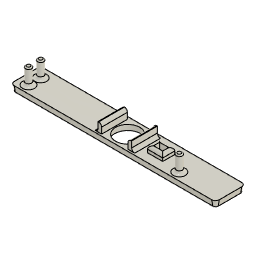
Front_Cover_OV5648_120DEG_AF v13 (Autodesk Fusion 360 design; units mm, degrees)
Autodesk Fusion 360 part; units mm, degrees
sketch "Sketch1" plane through (0, 0, 0) normal (0, 0, 1) x (1, 0, 0) in component "FrontCover"
  line L0 (0.9, 0) -> (66.1, 0)
  line L1 (67, 0.9) -> (67, 8.3)
  line L2 (66.1, 9.2) -> (0.9, 9.2)
  line L3 (0, 8.3) -> (0, 0.9)
  arc A0 (0.9, 9.2) -> (0, 8.3) centre (0.9, 8.3) ccw
  arc A1 (67, 8.3) -> (66.1, 9.2) centre (66.1, 8.3) ccw
  arc A2 (66.1, 0) -> (67, 0.9) centre (66.1, 0.9) ccw
  arc A3 (0, 0.9) -> (0.9, 0) centre (0.9, 0.9) ccw
  point P0 (67, 0)
  point P1 (0, 9.2)
  dimension "d1" = 67
  dimension "d2" = 9.2
  dimension "d3" = 0.9
  constraint horizontal L0
  constraint vertical L1
  constraint horizontal L2
  constraint vertical L3
  constraint coincident P1 L2
  constraint coincident P1 L3
  constraint tangent L2 A0
  constraint tangent L3 A0
  constraint tangent L1 A1
  constraint tangent L2 A1
  constraint equal A0 A1
  constraint coincident P0 L0
  constraint coincident P0 L1
  constraint tangent L0 A2
  constraint tangent L1 A2
  constraint equal A0 A2
  constraint coincident origin L0
  constraint coincident origin L3
  constraint tangent L0 A3
  constraint tangent L3 A3
  constraint equal A0 A3
  measures "d1" distance of origin P0
  measures "d2" distance of origin P1
  measures "d3" radius of A0
extrude "Extrude1" add sketch "Sketch1" along normal blind 2 draft 10 in component "FrontCover"
sketch "Sketch2" plane through (0, 0, 2) normal (0, 0, 1) x (-1, 0, 0) in component "FrontCover"
  line L0 (0.3527, -8.3) -> (0.3527, -0.9)
  arc A0 (0.3527, -0.9) -> (-0.9, 0.3527) centre (-0.9, -0.9) ccw
  line L1 (-0.9, 0.3527) -> (-66.1, 0.3527)
  arc A1 (-66.1, 0.3527) -> (-67.3527, -0.9) centre (-66.1, -0.9) ccw
  line L2 (-67.3527, -0.9) -> (-67.3527, -8.3)
  arc A2 (-67.3527, -8.3) -> (-66.1, -9.5527) centre (-66.1, -8.3) ccw
  line L3 (-66.1, -9.5527) -> (-0.9, -9.5527)
  arc A3 (-0.9, -9.5527) -> (0.3527, -8.3) centre (-0.9, -8.3) ccw
  line L4 (-66.1, -9.2) -> (-0.9, -9.2)
  arc A4 (-0.9, -9.2) -> (0, -8.3) centre (-0.9, -8.3) ccw
  line L5 (0, -8.3) -> (0, -0.9)
  arc A5 (0, -0.9) -> (-0.9, 0) centre (-0.9, -0.9) ccw
  line L6 (-0.9, 0) -> (-66.1, 0)
  arc A6 (-66.1, 0) -> (-67, -0.9) centre (-66.1, -0.9) ccw
  line L7 (-67, -0.9) -> (-67, -8.3)
  arc A7 (-67, -8.3) -> (-66.1, -9.2) centre (-66.1, -8.3) ccw
  line L8 (-1, -9.2) -> (-1, 0) construction
  circle A8 centre (-3, -6.25) radius 1
  circle A9 centre (-3, -2.25) radius 1
  circle A10 centre (-33.5, -4.5) radius 4
  circle A11 centre (-52.8, -2.25) radius 1
  line L9 (-37.85, -8.75) -> (-37.85, -0.25)
  line L10 (-29.15, -0.25) -> (-29.15, -8.75)
  line L11 (-29.15, -8.75) -> (-37.85, -0.25) construction
  line L12 (-37.85, -8.75) -> (-29.15, -0.25) construction
  line L13 (-27.95, -0.25) -> (-27.95, -8.75)
  line L14 (-39.05, -8.75) -> (-39.05, -0.25)
  line L15 (-37.85, -8.75) -> (-39.05, -8.75)
  line L16 (-37.85, -0.25) -> (-39.05, -0.25)
  line L17 (-29.15, -0.25) -> (-27.95, -0.25)
  line L18 (-29.15, -8.75) -> (-27.95, -8.75)
  line L19 (-46.05, -3.5) -> (-43.05, -3.5)
  line L20 (-43.05, -3.5) -> (-43.05, -5.5)
  line L21 (-43.05, -5.5) -> (-46.05, -5.5)
  line L22 (-46.05, -5.5) -> (-46.05, -3.5)
  line L23 (-46.05, -3.5) -> (-43.05, -5.5) construction
  line L24 (-43.05, -3.5) -> (-46.05, -5.5) construction
  line L25 (-42.05, -2.5) -> (-42.05, -6.5)
  line L26 (-42.05, -6.5) -> (-47.05, -6.5)
  line L27 (-47.05, -6.5) -> (-47.05, -2.5)
  line L28 (-47.05, -2.5) -> (-42.05, -2.5)
  point P0 (-33.5, -4.5)
  point P1 (-44.55, -4.5)
  dimension "d6" = 1
  dimension "d7" = 2
  dimension "d8" = 2
  dimension "d9" = 2
  dimension "d10" = 2
  dimension "d11" = 8
  dimension "d12" = 32.5
  dimension "d13" = 4.5
  dimension "d14" = 2.25
  dimension "d15" = 6.25
  dimension "d16" = 2
  dimension "d17" = 2.25
  dimension "d18" = 51.8
  dimension "d19" = 8.7
  dimension "d20" = 8.5
  dimension "d21" = -1.2
  dimension "d22" = -1.2
  dimension "d23" = 3
  dimension "d24" = 2
  dimension "d25" = 11.05
  dimension "d44" = -1
  constraint coincident L4 L8.start
  constraint coincident L6 L8.end
  constraint perpendicular L6 L8
  constraint parallel L9 L10
  constraint coincident L11 P0
  constraint coincident L12 P0
  constraint coincident P0 A10.centre
  constraint horizontal L19
  constraint perpendicular L19 L20
  constraint parallel L19 L21
  constraint parallel L20 L22
  constraint coincident L23 P1
  constraint coincident L24 P1
  measures "d6" distance of L5 L8
  measures "d7" diameter of A8
  measures "d8" distance of L8 A8.centre
  measures "d9" diameter of A9
  measures "d10" distance of L8 A9.centre
  measures "d11" diameter of A10
  measures "d12" distance of L8 P0
  measures "d13" distance of L6 P0
  measures "d14" distance of L6 A9.centre
  measures "d15" distance of L6 A8.centre
  measures "d16" diameter of A11
  measures "d17" distance of L6 A11.centre
  measures "d18" distance of L8 A11.centre
  measures "d19" distance of L9.end L10.start
  measures "d20" distance of L9.start L9.end
  measures "d23" distance of L20.end L21.end
  measures "d24" distance of L19.end L20.end
  measures "d25" distance of P0 P1
extrude "Extrude2" add sketch "Sketch2" along normal blind 3 contours L9 L14 L15 L16 in component "FrontCover"
extrude "Extrude3" add sketch "Sketch2" along normal blind 3 contours L10 L13 L17 L18 in component "FrontCover"
extrude "Extrude4" add sketch "Sketch2" along normal blind 5.5 contours A8 | A9 | A11 in component "FrontCover"
extrude "Extrude8" add sketch "Sketch2" along normal blind 2 contours L25 L26 L27 L28 in component "FrontCover"
extrude "Extrude5" cut sketch "Sketch2" against normal up to surface (2 mm away) draft 10 contours L19 L20 L21 L22 in component "FrontCover"
extrude "Extrude6" cut sketch "Sketch2" against normal up to surface (2 mm away) draft 10 contours A10 in component "FrontCover"
fillet "Fillet1" radius 1 11 edges at (3.9323, 1.8884, 2) (3.9323, 5.8884, 2) (53.7323, 1.8884, 2) (39.05, 4.5, 2) (27.95, 4.5, 2) (29.15, 4.5, 5) (37.85, 4.5, 5) (42.05, 4.5, 4) (47.05, 4.5, 4) (44.55, 2.5, 4) (44.55, 6.5, 4) in component "FrontCover"
fillet "Fillet3" radius 2 4 edges at (44.55, 3.1473, 0) (42.6973, 4.5, 0) (44.55, 5.8527, 0) (46.4027, 4.5, 0) in component "FrontCover"
fillet "Fillet4" radius 0.4 3 edges at (53.7323, 2.6116, 7.5) (3.9323, 6.6116, 7.5) (3.9323, 2.6116, 7.5) in component "FrontCover"
sketch "Sketch3" plane through (0, 0, 0) normal (0, 0, -1) x (1, 0, 0) in component "FrontCover"
  line L0 (66.1, 0) -> (0.9, 0)
  arc A0 (0.9, 0) -> (0, -0.9) centre (0.9, -0.9) ccw
  line L1 (0, -0.9) -> (0, -8.3)
  arc A1 (0, -8.3) -> (0.9, -9.2) centre (0.9, -8.3) ccw
  line L2 (0.9, -9.2) -> (66.1, -9.2)
  line L3 (19.8902, -2.6422) -> (16.4262, -0.642)
  line L4 (12.962, -2.6418) -> (12.9618, -6.6418)
  line L5 (14.926, -4.6419) -> (13.9261, -4.6418)
  line L6 (16.201, -2.434) -> (14.926, -4.6419)
  line L7 (17.2009, -2.434) -> (18.2009, -2.4341)
  line L8 (14.6511, -6.8499) -> (17.2009, -2.434)
  line L9 (16.4262, -0.642) -> (12.962, -2.6418)
  line L10 (18.2009, -2.4341) -> (15.6511, -6.8499)
  line L11 (13.9261, -4.6418) -> (15.201, -2.4339)
  line L12 (15.201, -2.4339) -> (16.201, -2.434)
  line L13 (18.9259, -4.6421) -> (17.651, -6.85)
  line L14 (15.6511, -6.8499) -> (14.6511, -6.8499)
  line L15 (17.651, -6.85) -> (16.651, -6.85)
  line L16 (17.926, -4.6421) -> (18.9259, -4.6421)
  line L17 (16.651, -6.85) -> (17.926, -4.6421)
  line L18 (12.9618, -6.6418) -> (16.4258, -8.642)
  line L19 (19.89, -6.6422) -> (19.8902, -2.6422)
  line L20 (16.4258, -8.642) -> (19.89, -6.6422)
  arc A2 (66.1, -9.2) -> (67, -8.3) centre (66.1, -8.3) ccw
  line L21 (67, -8.3) -> (67, -0.9)
  arc A3 (67, -0.9) -> (66.1, 0) centre (66.1, -0.9) ccw
  circle A4 centre (33.5, -4.5) radius 4.3527
  line L22 (41.0191, -7.5309) -> (41.0191, -1.4691)
  line L23 (41.0191, -1.4691) -> (48.0809, -1.4691)
  line L24 (48.0809, -1.4691) -> (48.0809, -7.5309)
  line L25 (48.0809, -7.5309) -> (41.0191, -7.5309)
extrude "Extrude7" cut sketch "Sketch3" against normal blind 0.5 contours L3 L4 L9 L18 L19 L20 in component "FrontCover"
component "FrontCover" placed x (1, 0, 0) y (0, 1, 0) z (0, 0, 1) at (0, 0, 0)
equation "d25 = ( ( 8.5 / 2 ) * 1 mm ) + 6.8 mm"
